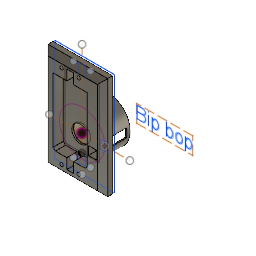
Servohholder (Autodesk Fusion 360 design; units mm, degrees)
Autodesk Fusion 360 part; units mm, degrees
sketch "Sketch1" plane through (0, 0, 0) normal (0, 1, 0) x (1, 0, 0)
  circle A0 centre (0, 0) radius 13.25
  dimension "d1" = 26.5
  measures "d1" diameter of A0
extrude "Extrude1" add sketch "Sketch1" along normal blind 15 makes body 1
sketch "Sketch2" plane through (0, 0, 0) normal (0, 0, 1) x (1, 0, 0)
  circle A0 centre (0.132, 10.5) radius 2.35
  dimension "d5" = 4.7
  dimension "d10" = 10.5
  measures "d5" diameter of A0
  measures "d10" distance of origin
extrude "Extrude2" add sketch "Sketch2" along normal blind 15 bodies 1
sketch "Sketch3" plane through (0, 0, 0) normal (0, 1, 0) x (1, 0, 0)
  circle A0 centre (0, 0) radius 12.5
  dimension "d8" = 25
  measures "d8" diameter of A0
extrude "Extrude3" cut sketch "Sketch3" along normal through all bodies 1
sketch "Sketch4" plane through (0, 0, 0) normal (0, 1, 0) x (1, 0, 0)
  line L0 (-16, -39.1044) -> (19, -39.1044)
  line L1 (19, 20.8956) -> (-16, 20.8956)
  line L2 (-16, 20.8956) -> (-16, -39.1044)
  line L3 (15.75, -2.5252) -> (10.75, -2.5252)
  line L4 (10.75, -2.5252) -> (10.75, 2.4748)
  line L5 (10.75, 2.4748) -> (15.75, 2.4748)
  line L6 (15.75, 2.4748) -> (15.75, -2.5252)
  line L7 (15.75, -2.5252) -> (10.75, 2.4748) construction
  line L8 (10.75, -2.5252) -> (15.75, 2.4748) construction
  circle A0 centre (0, 0) radius 13.25
  line L9 (19, 20.8956) -> (19, -39.1044)
  line L10 (32, -21) -> (64.7832, -21) construction
  line L11 (64.7832, -21) -> (64.7832, -31) construction
  line L12 (64.7832, -31) -> (32, -31) construction
  line L13 (32, -31) -> (32, -21) construction
  line L14 (0, -45) -> (0, 21) construction
  circle A1 centre (-5, 15) radius 1
  circle A2 centre (5, 15) radius 1
  line L15 (-19, 0) -> (28, 0) construction
  circle A3 centre (-5, -34) radius 1
  circle A4 centre (5, -34) radius 1
  line L16 (-10, -29) -> (10, -29)
  line L17 (10, -29) -> (10, 10)
  line L18 (10, 10) -> (-10, 10)
  line L19 (-10, 10) -> (-10, -29)
  circle A5 centre (0, 0) radius 5
  line L20 (-1.9268, -29) -> (2, -29)
  line L21 (2, -29) -> (2, -35)
  line L22 (2, -35) -> (-1.9268, -35)
  line L23 (-1.9268, -35) -> (-1.9268, -29)
  line L24 (-1.9609, 10) -> (2, 10)
  line L25 (2, 10) -> (2, 16)
  line L26 (2, 16) -> (-1.9609, 16)
  line L27 (-1.9609, 16) -> (-1.9609, 10)
  dimension "d13" = 5
  dimension "d14" = 5
  dimension "d15" = 2
  dimension "d16" = 49
  dimension "d23" = 35
  dimension "d24" = 60
  dimension "d25" = 39
  dimension "d26" = 20
  dimension "d27" = 10
  dimension "d28" = 10
  dimension "d29" = 10
  measures "d15" diameter of A3
  measures "d27" distance of A0.centre
  measures "d28" distance of A0.centre L17
  measures "d29" diameter of A5
extrude "Extrude11" add sketch "Sketch4" against normal blind 7 separate body contours L0 L1 L2 L9 | L3 L4 L5 A0 L17 | A0 L19 | A0 L17 L18 | A0 L18 L19 | A0 L18 L25 | A0 L18 L27 makes body 2
extrude "Extrude10" add sketch "Sketch4" against normal blind 1 contours L0 L1 L2 L9 | L3 L4 L5 A0 L17 | A0 L16 L17 L19 L20 | A0 L17 L18 L19 L24 | A0 L19 | A0 L17 L18 | A0 L18 L19 | L16 L20 L21 L22 L23 | A0 L18 L25 | A0 L18 L27 | A0 L18 L24 L25 L27 | A0 L25 L26 L27 bodies 2 1
extrude "Extrude12" cut sketch "Sketch4" along normal blind 13 contours L3 L5 L6 A0 | L3 L4 L5 A0 bodies 2
chamfer "Chamfer1" distance 3 angle 45 4 edges at (-16, -7, 9.1044) (1.5, -7, 39.1044) (19, -7, 9.1044) (1.5, -7, -20.8956) on bodies 2
chamfer "Chamfer2" distance 1 angle 45 4 edges at (19, 0, 9.1044) (1.5, 0, 39.1044) (-16, 0, 9.1044) (1.5, 0, -20.8956) on bodies 2
